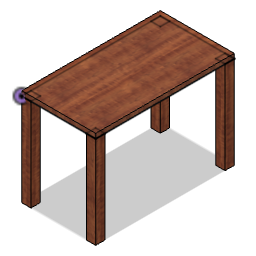
Table v5 (Autodesk Fusion 360 design; units mm, degrees)
Autodesk Fusion 360 part; units mm, degrees
sketch "Sketch1" plane through (0, 0, 0) normal (0, 1, 0) x (-1, 0, 0)
  line L0 (0, 0) -> (-1500, 0)
  line L1 (-1500, 0) -> (-1500, 800)
  line L2 (-1500, 800) -> (0, 800)
  line L3 (0, 800) -> (0, 0)
  line L4 (-1400, 800) -> (-1500, 800)
  line L5 (-1500, 800) -> (-1500, 700)
  line L6 (-1500, 700) -> (-1400, 700)
  line L7 (-1400, 700) -> (-1400, 800)
  line L8 (0, 800) -> (-100, 800)
  line L9 (-100, 800) -> (-100, 700)
  line L10 (-100, 700) -> (0, 700)
  line L11 (0, 700) -> (0, 800)
  line L12 (0, 0) -> (-100, 0)
  line L13 (-100, 0) -> (-100, 100)
  line L14 (-100, 100) -> (0, 100)
  line L15 (0, 100) -> (0, 0)
  line L16 (-1500, 0) -> (-1400, 0)
  line L17 (-1400, 0) -> (-1400, 100)
  line L18 (-1400, 100) -> (-1500, 100)
  line L19 (-1500, 100) -> (-1500, 0)
  dimension "d1" = 1500
  dimension "d2" = 800
  dimension "d3" = 100
  dimension "d4" = 100
  dimension "d5" = 100
  dimension "d6" = 100
  dimension "d7" = 100
  dimension "d8" = 100
  dimension "d9" = 100
  dimension "d10" = 100
  constraint horizontal L0
  constraint vertical L1
  constraint horizontal L2
  constraint vertical L3
  constraint coincident L0.start L3.end
  constraint horizontal L4
  constraint vertical L5
  constraint horizontal L6
  constraint vertical L7
  constraint coincident L2 L4.start
  constraint collinear L1 L5
  constraint horizontal L8
  constraint vertical L9
  constraint horizontal L10
  constraint vertical L11
  constraint horizontal L12
  constraint vertical L13
  constraint horizontal L14
  constraint vertical L15
  constraint horizontal L16
  constraint vertical L17
  constraint horizontal L18
  constraint vertical L19
  measures "d1" distance of L0.start L0.end
  measures "d2" distance of L0.start L2.end
  measures "d3" distance of L4.start L1.end
  measures "d4" distance of L4.start L6.end
  measures "d5" distance of L2.end L8.end
  measures "d6" distance of L2.end L10.end
  measures "d7" distance of L0.start L12.end
  measures "d8" distance of L0.start L14.end
  measures "d9" distance of L0.end L16.end
  measures "d10" distance of L0.end L18.end
extrude "Extrude1" add sketch "Sketch1" along normal blind 50
extrude "Extrude2" add sketch "Sketch1" against normal blind 1000 contours L0 L3 L12 L13 L14 L15 | L0 L1 L16 L17 L18 L19 | L2 L3 L8 L9 L10 L11 | L1 L2 L4 L5 L6 L7
named bodies: "Table"
